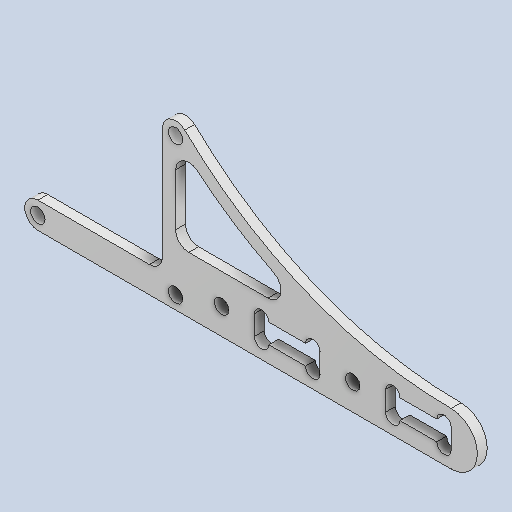
# Autodesk Inventor part: 3304_tesaki
Saved by Autodesk Inventor 2024 (Build 280153000, 153)
## iProperties
Created: 2024-01-03
Part Number: 3304_tesaki
Material: アルミニウム 2014-T4
Document SubType Name: Modeling
Designer: right
Density: 2.8 g/cm^3
Appearance: サテン
Mass: 2.12371 g
Surface Area: 14.7959 cm^2
Volume: 0.758467 cm^3
Author: right
Autodesk Inventor part; units mm, degrees
ref_plane "YZ Plane" through (0, 0, 0) normal (1, 0, 0) x (0, 1, 0)
ref_plane "XZ Plane" through (0, 0, 0) normal (0, 1, 0) x (-1, 0, 0)
ref_plane "XY Plane" through (0, 0, 0) normal (0, 0, 1) x (1, 0, 0)
sketch "スケッチ1" plane through (0, 0, 0) normal (0, 0, 1) x (1, 0, 0)
  circle A0 centre (-3.9908, -3.6656) radius 1 projected
  circle A1 centre (-24.9908, -24.6656) radius 1 projected
  line L0 (-3.9908, -3.6656) -> (-24.9908, -3.6656) construction
  line L1 (-24.9908, -3.6656) -> (-24.9908, -24.6656) construction
  line L2 (-24.9908, -24.6656) -> (-3.9908, -24.6656) construction
  line L3 (-3.9908, -24.6656) -> (-3.9908, -3.6656) construction
  circle A2 centre (-3.9908, -3.6656) radius 1.1
  circle A3 centre (-24.9908, -3.6656) radius 1.1
  circle A4 centre (-3.9908, -24.6656) radius 1.1
  circle A5 centre (-24.9908, -24.6656) radius 1.1
  circle A6 centre (-24.9908, -14.1656) radius 8 projected
  circle A7 centre (-24.9908, -24.6656) radius 2
  circle A8 centre (-3.9908, -24.6656) radius 2
  circle A9 centre (-24.9908, -3.6656) radius 2
  circle A10 centre (-3.9908, -3.6656) radius 2
  line L4 (-24.9908, -26.6656) -> (-1.9908, -26.6656)
  line L5 (-3.9908, -26.6656) -> (-3.9908, -22.6656)
  line L6 (-3.9908, -22.6656) -> (-24.9908, -22.6656)
  line L7 (-24.9908, -22.6656) -> (-24.9908, -26.6656)
  line L8 (-5.9908, -24.6656) -> (-1.9908, -24.6656)
  line L9 (-1.9908, -24.6656) -> (-1.9908, -3.6656)
  line L10 (-1.9908, -3.6656) -> (-5.9908, -3.6656)
  line L11 (-5.9908, -3.6656) -> (-5.9908, -24.6656)
  line L12 (18.0092, -24.1656) -> (8.0092, -24.1656)
  line L13 (8.0092, -24.1656) -> (8.0092, -21.1656)
  line L14 (8.0092, -21.1656) -> (18.0092, -21.1656)
  line L15 (18.0092, -21.1656) -> (18.0092, -24.1656)
  line L16 (38.0092, -24.1656) -> (28.0092, -24.1656)
  line L17 (28.0092, -24.1656) -> (28.0092, -21.1656)
  line L18 (28.0092, -21.1656) -> (38.0092, -21.1656)
  line L19 (38.0092, -21.1656) -> (38.0092, -24.1656)
  circle A11 centre (16.9092, -24.1656) radius 1.1
  line L20 (13.0092, -24.1656) -> (13.0092, -21.1656) construction
  line L21 (13.0092, -22.6656) -> (18.0092, -22.6656) construction
  line L22 (28.0092, -22.6656) -> (18.0092, -22.6656) construction
  line L23 (23.0092, -22.6656) -> (23.0092, -26.0364) construction
  circle A12 centre (9.1092, -24.1656) radius 1.1
  circle A13 centre (16.9092, -21.1656) radius 1.1
  circle A14 centre (9.1092, -21.1656) radius 1.1
  circle A15 centre (29.1092, -24.1656) radius 1.1
  circle A16 centre (36.9092, -24.1656) radius 1.1
  circle A17 centre (29.1092, -21.1656) radius 1.1
  circle A18 centre (36.9092, -21.1656) radius 1.1
  line L24 (42.0092, -26.6656) -> (-1.9908, -26.6656)
  line L25 (-1.9908, -26.6656) -> (-1.9908, -18.1656)
  line L26 (-1.9908, -18.1656) -> (42.0092, -18.1656)
  line L27 (42.0092, -18.1656) -> (42.0092, -26.6656)
  circle A19 centre (38.0092, -22.6656) radius 4
  arc A20 (-2.5997, -2.2287) -> (38.0092, -18.6656) centre (38.0092, 39.7168) ccw
  circle A21 centre (23.0092, -22.6656) radius 1.1
  circle A22 centre (3.0092, -22.6656) radius 1.1
  line L28 (38.0092, -18.6656) -> (-1.9908, -18.6656) construction
  point P0 (0, 0)
  point P1 (38.0092, -26.6656)
  point P2 (-5.9908, -22.6656)
  point P3 (15.8092, -24.1656)
  point P4 (10.2092, -24.1656)
  point P5 (10.2092, -21.1656)
  point P6 (15.8092, -21.1656)
  point P7 (35.8092, -21.1656)
  point P8 (35.8092, -24.1656)
  point P9 (30.2092, -24.1656)
  point P10 (30.2092, -21.1656)
  point P11 (30.3847, -18.1656)
  point P12 (42.0092, -22.6656)
  dimension "d11" = 4
  dimension "d24" = 2.2
  dimension "d0" = 21
  dimension "d1" = 21
  dimension "d2" = 2.2
  dimension "d5" = 21
  dimension "d8" = 21
  dimension "d14" = 21
  dimension "d17" = 21
  dimension "d20" = 10
  dimension "d21" = 3
  dimension "d22" = 10
  dimension "d23" = 3
  dimension "d25" = 2.5
  dimension "d26" = 3
  dimension "d28" = 10
  dimension "d29" = 10
  dimension "d31" = 2.2
  constraints: 58 end point, 17 centre point, 13 parallel, 9 horizontal, 8 symmetric about line, 7 midpoint, 7 point on line, 6 perpendicular, 6 point on circle, 4 tangent, 4 vertical, 3 coincident, 2 horizontal alignment, 1 line through centre, 29 other
  measures "d0" distance of L0.start L0.end
  measures "d1" distance of L0.end L1.end
  measures "d2" diameter of A2
  measures "d5" distance of A2.centre A3.centre
  measures "d8" distance of A2.centre A4.centre
  measures "d14" distance of point (-24.991, -24.666) A8.centre
  measures "d17" distance of point (-24.991, -24.666) A9.centre
  measures "d20" distance of L13.end L14.end
  measures "d21" distance of L12.end L13.end
  measures "d22" distance of L17.end L18.end
  measures "d23" distance of L16.end L17.end
  measures "d25" distance from line of L24 A12.centre
  measures "d26" distance from line of L26 A17.centre
  measures "d28" distance between parallel lines of L9 L13
  measures "d29" distance between parallel lines of L15 L17
  measures "d31" diameter of A21
extrude "押し出し1" add sketch "スケッチ1" along normal blind 1.5 contours L10 A10 A2 | A2 L10 A10 | L9 A8 L6 L11 A10 | A10 A20 L26 L9 | L26 A20 A19 L18 A17 L17 A15 L16 L24 L25 L9 | L11 A8 L4 A7 L6 | L6 A8 L11 | L8 A4 L5 A8 | L25 L4 A8 | A8 L5 A4 L8 | L5 A4 L8 A8 | L7 A5 A7 | A7 L7 A5 | L8 A4 L5 A8 | A19 L16 A16 L19 A18 L18 picked at (39.3425, -22.6656)
fillet "フィレット1" radius 2 1 edges at (-5.9908, -22.6656, 0.75)
sketch "スケッチ2" plane through (0, 0, 1.5) normal (0, 0, 1) x (1, 0, 0)
  line L0 (-24.9908, -26.6656) -> (38.0092, -26.6656) projected
  arc A0 (38.0092, -26.6656) -> (38.0092, -18.6656) centre (38.0092, -22.6656) ccw projected
  arc A1 (-2.5997, -2.2287) -> (38.0092, -18.6656) centre (38.0092, 39.7168) ccw projected
  arc A2 (-2.5997, -2.2287) -> (-5.9908, -3.6656) centre (-3.9908, -3.6656) ccw projected
  line L1 (-5.9908, -3.6656) -> (-5.9908, -20.6656) projected
  arc A3 (-7.9908, -22.6656) -> (-5.9908, -20.6656) centre (-7.9908, -20.6656) ccw projected
  line L2 (-7.9908, -22.6656) -> (-24.9908, -22.6656) projected
  arc A4 (-24.9908, -22.6656) -> (-24.9908, -26.6656) centre (-24.9908, -24.6656) ccw projected
  circle A5 centre (-24.9908, -24.6656) radius 1.1 projected
  circle A6 centre (-3.9908, -3.6656) radius 1.1 projected
  circle A7 centre (-3.9908, -24.6656) radius 1.1 projected
  line L3 (18.0092, -21.1656) -> (18.0092, -24.1656) projected
  arc A8 (15.8092, -24.1656) -> (18.0092, -24.1656) centre (16.9092, -24.1656) ccw projected
  line L4 (15.8092, -24.1656) -> (10.2092, -24.1656) projected
  arc A9 (8.0092, -24.1656) -> (10.2092, -24.1656) centre (9.1092, -24.1656) ccw projected
  line L5 (8.0092, -24.1656) -> (8.0092, -21.1656) projected
  arc A10 (10.2092, -21.1656) -> (8.0092, -21.1656) centre (9.1092, -21.1656) ccw projected
  line L6 (10.2092, -21.1656) -> (15.8092, -21.1656) projected
  arc A11 (18.0092, -21.1656) -> (15.8092, -21.1656) centre (16.9092, -21.1656) ccw projected
  circle A12 centre (3.0092, -22.6656) radius 1.1 projected
  circle A13 centre (23.0092, -22.6656) radius 1.1 projected
  line L7 (30.2092, -21.1656) -> (35.8092, -21.1656) projected
  arc A14 (38.0092, -21.1656) -> (35.8092, -21.1656) centre (36.9092, -21.1656) ccw projected
  line L8 (38.0092, -21.1656) -> (38.0092, -24.1656) projected
  arc A15 (35.8092, -24.1656) -> (38.0092, -24.1656) centre (36.9092, -24.1656) ccw projected
  line L9 (35.8092, -24.1656) -> (30.2092, -24.1656) projected
  arc A16 (28.0092, -24.1656) -> (30.2092, -24.1656) centre (29.1092, -24.1656) ccw projected
  line L10 (28.0092, -24.1656) -> (28.0092, -21.1656) projected
  arc A17 (30.2092, -21.1656) -> (28.0092, -21.1656) centre (29.1092, -21.1656) ccw projected
  line L11 (38.0092, -24.6656) -> (-7.9908, -24.6656)
  arc A18 (-7.9908, -24.6656) -> (-3.9908, -20.6656) centre (-7.9908, -20.6656) ccw
  line L12 (-3.9908, -16.0656) -> (-3.9908, -8.1535)
  arc A19 (-0.7084, -6.6187) -> (38.0092, -20.6656) centre (38.0092, 39.7168) ccw
  arc A20 (38.0092, -24.6656) -> (38.0092, -20.6656) centre (38.0092, -22.6656) ccw
  arc A21 (-0.7084, -6.6187) -> (-3.9908, -8.1535) centre (-1.9908, -8.1535) ccw
  line L13 (20.4813, -18.0656) -> (-1.9908, -18.0656)
  arc A22 (-3.9908, -16.0656) -> (-1.9908, -18.0656) centre (-1.9908, -16.0656) ccw
  point P0 (0, 0)
  point P1 (-3.9908, -3.6656)
  point P2 (17.4157, -17.0454)
  point P3 (-3.9908, -15.0454)
  point P4 (9.1092, -20.0656)
  point P5 (9.2452, -18.0656)
  dimension "d35" = 2
  dimension "d36" = 2
  dimension "d40" = 2
  dimension "d41" = 2
  constraints: 14 point on circle, 6 end point, 5 centre point, 4 tangent, 3 point on line, 1 horizontal, 1 midpoint, 4 other
  measures "d35" distance between parallel lines of L0 L11
  measures "d36" radius of A21
  measures "d40" vertical distance of point (9.109, -20.066) point (9.245, -18.066)
  measures "d41" radius of A22
extrude "押し出し2" cut sketch "スケッチ2" against normal blind 1.5 contours L13 A22 L12 A21 A19
fillet "フィレット2" [suppressed]
fillet "フィレット3" radius 2 1 edges at (20.4813, -18.0656, 0.75)
equation "\"d5\" = d0"
equation "\"d8\" = d1"
equation "\"d14\" = d0"
equation "\"d17\" = d8"
